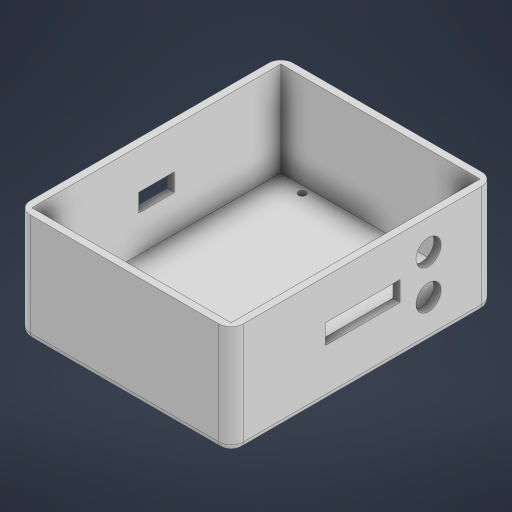
# Autodesk Inventor part: base
Saved by Autodesk Inventor 2024 (Build 280153000, 153)
## iProperties
Created: 2023-07-23
Part Number: base
Material: Generic
Document SubType Name: Modeling
Designer: Noah
Density: 1 g/cm^3
Appearance: Default
Author: Noah
## iProperties of the stored document base_3DPrint.ipt
Created: 2023-07-30
Part Number: base_3DPrint
Material: Generic
Document SubType Name: Modeling
Designer: Noah
Density: 1 g/cm^3
Appearance: Default
Author: Noah
Autodesk Inventor part; units mm, degrees
ref_plane "YZ Plane" through (0, 0, 0) normal (1, 0, 0) x (0, 1, 0)
ref_plane "XZ Plane" through (0, 0, 0) normal (0, 1, 0) x (-1, 0, 0)
ref_plane "XY Plane" through (0, 0, 0) normal (0, 0, 1) x (1, 0, 0)
sketch "Sketch1" plane through (0, 0, 0) normal (0, 1, 0) x (-1, 0, 0)
  line L0 (0, 0) -> (50, 0)
  line L1 (50, 0) -> (50, -70)
  line L2 (50, -70) -> (0, -70)
  line L3 (0, -70) -> (0, 0)
  line L4 (50, 0) -> (48, 0)
  line L5 (50, -2) -> (50, 0)
  circle A0 centre (48, -2) radius 1
  line L6 (25, 0) -> (25, -70)
  line L7 (50, -35) -> (0, -35)
  circle A1 centre (2, -2) radius 1
  circle A2 centre (48, -68) radius 1
  circle A3 centre (2, -68) radius 1
  line L8 (52, 2) -> (-2, 2)
  line L9 (-2, 2) -> (-2, -72)
  line L10 (-2, -72) -> (52, -72)
  line L11 (50, -35) -> (56, -35)
  line L12 (56, -35) -> (58, -35)
  line L13 (52, 2) -> (58, 2)
  line L14 (58, 2) -> (58, -72)
  line L15 (58, -72) -> (52, -72)
  line L16 (50, 0) -> (56, 0)
  line L17 (56, 0) -> (56, -70)
  line L18 (56, -70) -> (50, -70)
  line L19 (49.1547, 0) -> (50.3094, -2)
  line L20 (50.3094, -2) -> (49.1547, -4)
  line L21 (49.1547, -4) -> (46.8453, -4)
  line L22 (46.8453, -4) -> (45.6906, -2)
  line L23 (45.6906, -2) -> (46.8453, 0)
  line L24 (46.8453, 0) -> (49.1547, 0)
  line L25 (0.8453, 0) -> (-0.3094, -2)
  line L26 (-0.3094, -2) -> (0.8453, -4)
  line L27 (0.8453, -4) -> (3.1547, -4)
  line L28 (3.1547, -4) -> (4.3094, -2)
  line L29 (4.3094, -2) -> (3.1547, 0)
  line L30 (49.1547, -70) -> (50.3094, -68)
  line L31 (50.3094, -68) -> (49.1547, -66)
  line L32 (49.1547, -66) -> (46.8453, -66)
  line L33 (46.8453, -66) -> (45.6906, -68)
  line L34 (45.6906, -68) -> (46.8453, -70)
  line L35 (0.8453, -70) -> (-0.3094, -68)
  line L36 (-0.3094, -68) -> (0.8453, -66)
  line L37 (3.1547, -66) -> (4.3094, -68)
  line L38 (4.3094, -68) -> (3.1547, -70)
  line L39 (3.1547, -66) -> (0.8453, -66)
  dimension "d0" = 50
  dimension "d1" = 70
  dimension "d4" = 2
  dimension "d5" = 2
  dimension "d6" = 2
  dimension "d8" = 6
  dimension "d9" = 2
  constraints: 80 end point, 21 symmetric about line, 6 horizontal, 5 midpoint, 4 centre point, 4 perpendicular, 3 parallel, 1 coincident, 1 collinear, 1 point on line, 18 other
  measures "d0" distance of L1.end L2.end
  measures "d1" distance of L0.end L1.end
  measures "d4" distance from line of L0 A0.centre
  measures "d5" distance of L5.start A0.centre
  measures "d6" diameter of A0
  measures "d8" distance of L7.start L11.end
  measures "d9" distance of L11.end L12.end
extrude "Extrusion1" add sketch "Sketch1" along normal blind 40 contours L14 L15 L10 L9 L8 L13 | L3 L26 L25 | L3 L35 L36
extrude "Extrusion2" add sketch "Sketch1" against normal blind 2 contours L14 L15 L10 L9 L8 L13 | L0 L25 L3 | L0 L29 L28 L27 L26 L3 L25 | L3 L26 L25 | L0 L6 L7 L3 L26 L27 L28 L29 | L0 L23 L22 L21 L20 L1 L7 L6 | L7 L6 L2 L38 L37 L39 L36 L3 | L0 L19 L1 L20 L21 L22 L23 | L7 L1 L31 L32 L33 L34 L2 L6 | L36 L39 L37 L38 L2 L35 L3 | L3 L35 L36 | L11 L17 L18 L1 L30 L31 | L1 L20 L19 L16 L17 L11 | L35 L2 L3 | L0 L1 L19 | L34 L33 L32 L31 L1 L30 L2 | L1 L19 L20 | L31 L30 L1 | L30 L1 L2
sketch "Sketch2" plane through (0, -2, 0) normal (0, -1, 0) x (1, 0, 0)
  circle A0 centre (-2, -2) radius 1 projected
  line L0 (0.0173, -3.1247) -> (-1.9653, -4.3094)
  line L1 (-1.9653, -4.3094) -> (-3.9827, -3.1847)
  line L2 (-3.9827, -3.1847) -> (-4.0173, -0.8753)
  line L3 (-4.0173, -0.8753) -> (-2.0347, 0.3094)
  line L4 (-2.0347, 0.3094) -> (-0.0173, -0.8153)
  line L5 (-0.0173, -0.8153) -> (0.0173, -3.1247)
  circle A1 centre (-2, -68) radius 1 projected
  circle A2 centre (-48, -2) radius 1 projected
  circle A3 centre (-48, -68) radius 1 projected
  line L6 (-25, -68) -> (-25, 0)
  line L7 (0, -35) -> (-48, -35)
  circle A4 centre (-2, -68) radius 1
  line L8 (0.0173, -66.8753) -> (-1.9653, -65.6906)
  line L9 (-1.9653, -65.6906) -> (-3.9827, -66.8153)
  line L10 (-3.9827, -66.8153) -> (-4.0173, -69.1247)
  line L11 (-4.0173, -69.1247) -> (-2.0347, -70.3094)
  line L12 (-2.0347, -70.3094) -> (-0.0173, -69.1847)
  line L13 (-0.0173, -69.1847) -> (0.0173, -66.8753)
  circle A5 centre (-48, -2) radius 1
  line L14 (-50.0173, -3.1247) -> (-48.0347, -4.3094)
  line L15 (-48.0347, -4.3094) -> (-46.0173, -3.1847)
  line L16 (-46.0173, -3.1847) -> (-45.9827, -0.8753)
  line L17 (-45.9827, -0.8753) -> (-47.9653, 0.3094)
  line L18 (-47.9653, 0.3094) -> (-49.9827, -0.8153)
  line L19 (-49.9827, -0.8153) -> (-50.0173, -3.1247)
  line L20 (-49.9827, -69.1847) -> (-50.0173, -66.8753)
  line L21 (-50.0173, -66.8753) -> (-48.0347, -65.6906)
  line L22 (-48.0347, -65.6906) -> (-46.0173, -66.8153)
  line L23 (-47.9653, -70.3094) -> (-49.9827, -69.1847)
  line L24 (-45.9827, -69.1247) -> (-47.9653, -70.3094)
  line L25 (-46.0173, -66.8153) -> (-45.9827, -69.1247)
  line L26 (2, 2) -> (-58, 2) projected
  line L27 (-58, 2) -> (-58, -72) projected
  line L28 (-58, -72) -> (2, -72) projected
  line L29 (2, -72) -> (2, 2) projected
  circle A6 centre (-48, -2) radius 1 projected
  circle A7 centre (-2, -2) radius 1 projected
  circle A8 centre (-2, -68) radius 1 projected
  circle A9 centre (-48, -68) radius 1 projected
  point P0 (0, 0)
  point P1 (0, -1.97)
  point P2 (-25, -35)
  point P3 (0, -68.03)
  point P4 (-50, 0)
  point P5 (-50, -1.97)
  constraints: 52 end point, 21 symmetric about line, 2 centre point, 2 point on line, 1 coincident, 1 midpoint, 15 other
extrude "Extrusion3" add sketch "Sketch2" along normal blind 2 contours L29 L28 L27 L26
sketch "Sketch3" plane through (2, 40, 2) normal (1, 0, 0) x (0, 0, -1)
  line L0 (74, -44) -> (74, 0) projected
  line L1 (0, 0) -> (74, 0) projected
  line L2 (0, -44) -> (0, 0) projected
  line L3 (74, -44) -> (0, -44) projected
  line L4 (72, -40) -> (2, -40) projected
  line L5 (0, -40) -> (74, -40)
  line L6 (2, -40) -> (72, -40) projected
  line L7 (37, -27.5) -> (74, -27.5)
  line L8 (55.5, -27.5) -> (55.5, -22)
  line L9 (55.5, -27.5) -> (55.5, -33)
  circle A0 centre (55.5, -22) radius 3.5
  circle A1 centre (55.5, -33) radius 3.5
  line L10 (37, -27.5) -> (0, -27.5)
  line L11 (2.8687, -33.5508) -> (24.5082, -33.5508) construction
  line L12 (24.5082, -33.5508) -> (24.5082, -37.2201) construction
  line L13 (24.5082, -37.2201) -> (2.8687, -37.2201) construction
  line L14 (2.8687, -37.2201) -> (2.8687, -33.5508) construction
  line L15 (26.5, -30.25) -> (47.5, -30.25)
  line L16 (47.5, -30.25) -> (47.5, -24.75)
  line L17 (47.5, -24.75) -> (26.5, -24.75)
  line L18 (26.5, -24.75) -> (26.5, -30.25)
  line L19 (26.5, -30.25) -> (47.5, -24.75) construction
  line L20 (47.5, -30.25) -> (26.5, -24.75) construction
  dimension "d16" = 4
  dimension "d23" = 5.5
  dimension "d24" = 37
  dimension "d25" = 5.5
  dimension "d26" = 7
  dimension "d27" = 7
  constraints: 22 end point, 4 perpendicular, 4 point on line, 3 midpoint, 2 centre point, 2 coincident, 2 parallel, 2 vertical, 1 horizontal, 2 other
  measures "d16" distance from line of L3 L4.end
  measures "d23" distance of L8.start L9.end
  measures "d24" distance of L7.start L7.end
  measures "d25" distance of L8.start L8.end
  measures "d26" diameter of A0
  measures "d27" diameter of A1
extrude "Extrusion4" cut sketch "Sketch3" against normal blind 2 contours A1 | A0
fillet "Fillet2" radius 3.5 4 edges at (2, 18, 2) (2, 18, -72) (-58, 18, -72) (-58, 18, 2)
fillet "Fillet3" radius 1.75 8 edges at (0.9749, -4, 0.9749) (-28, -4, 2) (-56.9749, -4, 0.9749) (-58, -4, -35) (-56.9749, -4, -70.9749) (-28, -4, -72) (0.9749, -4, -70.9749) (2, -4, -35)
sketch "Sketch4" plane through (0, 40, 0) normal (0, 1, 0) x (1, 0, 0)
  line L0 (-65.2671, -10.9977) -> (8.3381, -10.9977)
  line L1 (8.3381, -10.9977) -> (8.3381, 80.2901)
  line L2 (8.3381, 80.2901) -> (-65.2671, 80.2901)
  line L3 (-65.2671, 80.2901) -> (-65.2671, -10.9977)
  point P0 (0, 0)
  constraints: 8 end point, 2 parallel, 1 horizontal, 1 perpendicular
extrude "Extrusion5" cut sketch "Sketch4" against normal blind 13.5
extrude "Extrusion6" cut sketch "Sketch3" against normal up to surface (2 mm away) contours L16 L15 L18 L10 L7 | L7 L10 L18 L17 L16
sketch "Sketch5" plane through (-58, -2.25, -68.5) normal (-1, 0, 0) x (0, 0, 1)
  line L0 (67, 0) -> (0, 0) projected
  line L1 (33.5, 0) -> (33.5, 17.5)
  line L2 (23, 17.5) -> (44, 17.5) projected
  line L3 (33.5, 17.5) -> (38.6471, 17.5) construction
  line L4 (33.5, 17.5) -> (38.5, 17.5)
  line L5 (38.5, 17.5) -> (38.5, 12.5)
  line L6 (38.5, 12.5) -> (28.5, 12.5)
  line L7 (28.5, 12.5) -> (28.5, 17.5)
  line L8 (38.5, 17.5) -> (28.5, 17.5)
  point P0 (68.5, 2.25)
  dimension "d39" = 17.5
  dimension "d42" = 5
  dimension "d43" = 5
  dimension "d44" = 10
  constraints: 14 end point, 3 perpendicular, 2 point on line, 1 horizontal, 1 midpoint, 1 vertical
  measures "d39" distance of L1.start L1.end
  measures "d42" distance of L1.end L4.end
  measures "d43" distance of L4.end L5.end
  measures "d44" distance of L5.end L6.end
extrude "Extrusion7" cut sketch "Sketch5" against normal up to surface (2 mm away)
body "Solid1"
